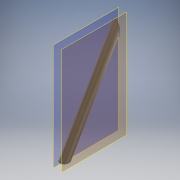
# Autodesk Inventor part: Pipe7
Saved by Autodesk Inventor 2018 (Build 220112000, 112)
## iProperties
Created: 2017-09-13
Part Number: Pipe7
Material: 鋼、炭素鋼
Document SubType Name: Modeling
Designer: mura5
Density: 7.85 g/cm^3
Appearance: 半つや出し
Author: mura5
Autodesk Inventor part; units mm, degrees
ref_plane "XZ Plane" through (0, 0, 0) normal (0, 1, 0) x (-1, 0, 0)
ref_plane "XY Plane" through (0, 0, 0) normal (0, 0, 1) x (1, 0, 0)
sketch "スケッチ1" plane through (0, 0, 0) normal (1, 0, 0) x (0, 1, 0)
  line L0 (0, 0) -> (-186.4, 0)
  line L1 (0, 0) -> (0, 326.4)
  line L2 (0, 326.4) -> (-186.4, 0)
  dimension "d0" = 186.4
  dimension "d1" = 326.4
  constraints: 6 end point, 1 horizontal, 1 vertical
  measures "d0" distance of L0.start L0.end
  measures "d1" distance of L0.start L1.end
ref_plane "作業平面1" through (0, -186.4, 0) normal (0, -0.4959097, -0.8683741) x (1, 0, 0)
sketch "スケッチ3" plane through (0, -186.4, 0) normal (0, -0.4959097, -0.8683741) x (1, 0, 0)
  circle A0 centre (0, -13.6) radius 13.6
  circle A1 centre (0, -13.6) radius 11.3
  point P0 (0, -161.8649)
  point P1 (0, 0)
  dimension "d4" = 27.2
  dimension "d5" = 13.6
  dimension "d6" = 2.3
  constraints: 2 centre point, 1 other
  measures "d4" diameter of A0
  measures "d5" distance of point (0, 0) A0.centre
  measures "d6" radial gap between concentric circles of A0 A1
extrude "押し出し1" add sketch "スケッチ3" against normal up to surface (375.8749 mm away)
extrude "押し出し2" cut sketch "スケッチ1" along normal mid plane 27.2 keep common part
ref_plane "作業平面2" through (-13.6, -174.5901, -6.7444) normal (-1, 0, 0) x (0, -1, 0)
ref_plane "作業平面3" through (13.6, -174.5901, -6.7444) normal (1, 0, 0) x (0, 1, 0)
sketch "スケッチ4" plane through (13.6, -174.5901, -6.7444) normal (1, 0, 0) x (0, 1, 0)
  line L0 (174.5901, 278.2957) -> (174.5901, 333.1444) construction
  line L1 (-11.8099, 6.7444) -> (19.513, 6.7444) construction
  line L2 (174.5901, 333.1444) -> (-11.8099, 6.7444) construction
  line L3 (174.5901, 278.2957) -> (19.513, 6.7444) construction
  line L4 (174.5901, 278.2957) -> (150.9703, 291.7844) construction
  line L5 (19.513, 6.7444) -> (-4.1068, 20.2331) construction
  line L6 (-11.8099, 6.7444) -> (174.5901, 333.1444) construction
  point P0 (174.5901, 6.7444)
  dimension "d11" = 375.8749
  dimension "d12" = 312.7124
  dimension "d13" = 27.2
  dimension "d14" = 29.73
  dimension "d15" = 60.27
  dimension "d16" = 47.6292
  dimension "d17" = 15.5333
  constraints: 8 end point, 2 perpendicular, 2 point on line
  measures "d11" distance of L0.end L1.start
  measures "d12" distance of L1.end L0.start
  measures "d13" distance between parallel lines of L2 L3
  measures "d14" angle of L2 L0
  measures "d15" angle of L2 L1
  measures "d16" distance from line of L0.end L4
  measures "d17" distance from line of L1.start L5
